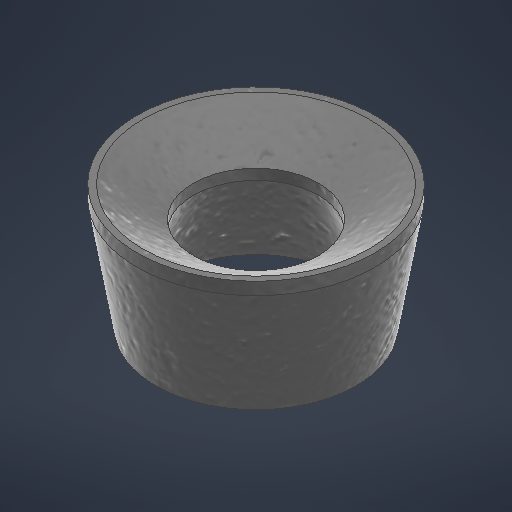
# Autodesk Inventor part: GRAFITO
Saved by Autodesk Inventor 2025 (Build 290162010, 162A)
## iProperties
Created: 2024-07-24
Part Number: GRAFITO
Material: Genérico
Document SubType Name: Modeling
Designer: hansm
Density: 1 g/cm^3
Appearance: Valor por defecto
Author: hansm
Autodesk Inventor part; units mm, degrees
ref_plane "YZ Plane" through (0, 0, 0) normal (1, 0, 0) x (0, 1, 0)
ref_plane "XZ Plane" through (0, 0, 0) normal (0, 1, 0) x (-1, 0, 0)
ref_plane "XY Plane" through (0, 0, 0) normal (0, 0, 1) x (1, 0, 0)
sketch "Boceto1" plane through (0, 0, 0) normal (0, 0, 1) x (1, 0, 0)
  line L0 (-24, 23.6746) -> (-21.5, 23.6746)
  line L1 (-28.5, 50.5) -> (-24, 23.6746)
  line L2 (-28.5, 50.5) -> (-28.5, 53.5)
  line L3 (-28.5, 53.5) -> (-27, 53.5)
  line L4 (-27, 53.5) -> (-15, 46.1746)
  line L5 (-15, 46.1746) -> (-15, 43.6746)
  line L6 (-15, 43.6746) -> (-21.5, 23.6746)
  line L7 (0, -10.7) -> (0, 64.2) projected
  point P0 (0, 0)
  dimension "d5" = 2.5
  dimension "d6" = 4.5
  dimension "d7" = 3
  dimension "d8" = 1.5
  dimension "d9" = 12
  dimension "d10" = 2.5
  dimension "d11" = 20
  constraints: 14 end point, 1 horizontal, 1 parallel, 1 perpendicular, 1 vertical
  measures "d5" distance of L0.start L0.end
  measures "d6" horizontal distance of L0.start L1.start
  measures "d7" distance of L1.start L2.end
  measures "d8" distance of L2.end L3.end
  measures "d9" horizontal distance of L4.end L3.end
  measures "d10" distance of L4.end L5.end
  measures "d11" vertical distance of L0.end L5.end
revolve "Revolución1" add sketch "Boceto1" angle 360 about axis through (0, -10, 0) along (0, 1, 0)
